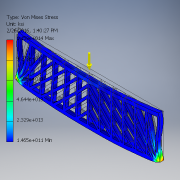
# Autodesk Inventor part: Haupt
Saved by Autodesk Inventor 2016 (Build 200138000, 138)
## iProperties
Created: 2016-02-25
Part Number: Haupt
Material: ABS Plastic
Document SubType Name: Modeling
Designer: 1750019
Density: 1.06 g/cm^3
Appearance: Smooth - White
Mass: 7.89342 g
Surface Area: 110.255 cm^2
Volume: 7.44663 cm^3
Author: 1750019
Autodesk Inventor part; units mm, degrees
ref_plane "YZ Plane" through (0, 0, 0) normal (1, 0, 0) x (0, 1, 0)
ref_plane "XZ Plane" through (0, 0, 0) normal (0, 1, 0) x (-1, 0, 0)
ref_plane "XY Plane" through (0, 0, 0) normal (0, 0, 1) x (1, 0, 0)
sketch "Sketch1" plane through (0, 0, 0) normal (0, 0, 1) x (1, 0, 0)
  line L0 (0, 0) -> (132.2917, 0) construction
  line L1 (132.2917, 0) -> (132.2917, -49.2125) construction
  line L2 (132.2917, -49.2125) -> (0, -49.2125) construction
  line L3 (0, -49.2125) -> (0, 0) construction
  line L4 (0, 0) -> (3.0776, 0) construction
  line L5 (3.0776, -2.3503) -> (3.0776, 0) construction
  line L6 (3.0776, -2.3503) -> (3.0776, -39.2903)
  line L7 (3.0776, -39.2903) -> (129.7257, -39.2903)
  line L8 (129.7257, -39.2903) -> (129.7257, -2.3503)
  line L9 (129.7257, -2.3503) -> (3.0776, -2.3503)
  line L10 (127.7764, -5.4053) -> (127.7764, -32.6911)
  line L11 (4.5608, -34.0848) -> (4.5608, -5.4053)
  line L12 (6.1422, -36.2512) -> (13.5226, -11.3064)
  line L13 (4.5608, -34.0848) -> (13.281, -5.4053)
  line L14 (57.0276, -34.9071) -> (65.3338, -26.3655)
  line L15 (58.4098, -36.2512) -> (65.3338, -29.1311)
  line L16 (127.7764, -32.6911) -> (119.3002, -5.4053)
  line L17 (119.3002, -12.0971) -> (126.3383, -36.2512)
  line L18 (74.4483, -36.2512) -> (67.1832, -28.7272)
  line L19 (75.8144, -34.9321) -> (67.1832, -25.9933)
  line L20 (4.5608, -5.4053) -> (13.281, -5.4053)
  line L21 (13.5226, -11.3064) -> (13.5226, -23.6805)
  line L22 (8.2509, -36.2512) -> (13.5226, -27.2721)
  line L23 (15.2246, -24.3731) -> (23.8802, -9.6304)
  line L24 (6.1422, -36.2512) -> (13.5226, -23.6805)
  line L25 (15.233, -20.7672) -> (23.8802, -6.0388)
  line L26 (8.2509, -36.2512) -> (13.5226, -29.8719)
  line L27 (10.6077, -36.2512) -> (13.5226, -32.7238)
  line L28 (13.5226, -36.2512) -> (10.6077, -36.2512)
  line L29 (17.7071, -36.2512) -> (23.8802, -29.7591)
  line L30 (23.8802, -36.2512) -> (23.8802, -29.7591)
  line L31 (25.4476, -28.1107) -> (25.4476, -36.2512)
  line L32 (15.1971, -36.2512) -> (23.8802, -27.1194)
  line L33 (23.8802, -36.2512) -> (17.7071, -36.2512)
  line L34 (25.569, -36.2512) -> (25.4476, -36.2512)
  line L35 (13.5226, -27.2721) -> (13.5226, -29.8719)
  line L36 (13.5226, -32.7238) -> (13.5226, -36.2512)
  line L37 (15.1971, -36.2512) -> (15.21, -30.6819)
  line L38 (15.2167, -27.8219) -> (15.2246, -24.3731)
  line L39 (15.233, -20.7672) -> (15.2686, -5.4053)
  line L40 (23.8802, -6.0388) -> (23.8802, -5.4053)
  line L41 (15.2686, -5.4053) -> (23.8802, -5.4053)
  line L42 (15.2167, -27.8219) -> (23.8802, -17.3381)
  line L43 (25.4476, -15.4414) -> (33.7411, -5.4053)
  line L44 (23.8802, -27.1194) -> (23.8802, -20.19)
  line L45 (23.8802, -17.3381) -> (23.8802, -9.6304)
  line L46 (25.4476, -5.4053) -> (25.4476, -15.4414)
  line L47 (25.4476, -18.2933) -> (25.4476, -25.471)
  line L48 (15.21, -30.6819) -> (23.8802, -20.19)
  line L49 (33.7411, -36.2512) -> (33.7411, -30.6389)
  line L50 (35.7136, -36.2512) -> (35.7136, -28.6156)
  line L51 (25.569, -36.2512) -> (33.7411, -27.8688)
  line L52 (28.2696, -36.2512) -> (33.7411, -30.6389)
  line L53 (33.7411, -36.2512) -> (28.2696, -36.2512)
  line L54 (33.7411, -27.8688) -> (33.7411, -19.3886)
  line L55 (33.7411, -16.7489) -> (33.7411, -8.2573)
  line L56 (25.4476, -25.471) -> (33.7411, -16.7489)
  line L57 (35.7136, -14.6745) -> (44.5272, -5.4053)
  line L58 (35.7136, -25.8455) -> (35.7136, -17.3142)
  line L59 (35.7136, -14.6745) -> (35.7136, -5.4053)
  line L60 (25.4476, -28.1107) -> (33.7411, -19.3886)
  line L61 (35.7136, -17.3142) -> (44.5272, -8.045)
  line L62 (25.4476, -18.2933) -> (33.7411, -8.2573)
  line L63 (25.4476, -5.4053) -> (33.7411, -5.4053)
  line L64 (35.7136, -5.4053) -> (44.5272, -5.4053)
  line L65 (35.7136, -25.8455) -> (44.5272, -16.805)
  line L66 (46.4045, -14.8793) -> (55.1798, -5.8781)
  line L67 (35.7136, -28.6156) -> (44.5272, -19.5751)
  line L68 (46.4045, -17.6495) -> (55.1798, -8.6483)
  line L69 (46.4045, -14.8793) -> (46.4045, -5.4053)
  line L70 (44.5272, -8.045) -> (44.5272, -16.805)
  line L71 (36.0978, -36.2512) -> (44.5272, -27.6711)
  line L72 (44.5272, -19.5751) -> (44.5272, -27.6711)
  line L73 (44.5272, -30.4311) -> (44.5272, -36.2512)
  line L74 (46.4045, -34.3207) -> (46.4045, -28.5054)
  line L75 (46.4045, -25.7602) -> (46.4045, -17.6495)
  line L76 (38.8531, -36.2512) -> (44.5272, -30.4311)
  line L77 (55.1798, -27.8779) -> (55.1798, -36.2512)
  line L78 (47.0372, -36.2512) -> (55.1798, -27.8779)
  line L79 (57.0276, -25.9778) -> (65.3338, -17.4362)
  line L80 (57.0276, -25.9778) -> (57.0276, -34.9071)
  line L81 (46.4045, -34.3207) -> (55.1798, -25.2968)
  line L82 (57.0276, -23.3967) -> (65.3338, -14.8551)
  line L83 (44.5272, -36.2512) -> (38.8531, -36.2512)
  line L84 (36.0978, -36.2512) -> (35.7136, -36.2512)
  line L85 (55.1798, -36.2512) -> (47.0372, -36.2512)
  line L86 (65.3338, -36.2512) -> (58.4098, -36.2512)
  line L87 (65.3338, -29.1311) -> (65.3338, -36.2512)
  line L88 (67.1832, -28.7272) -> (67.1832, -36.2512)
  line L89 (65.3338, -17.4362) -> (65.3338, -26.3655)
  line L90 (67.1832, -17.0999) -> (67.1832, -25.9933)
  line L91 (55.1798, -8.6483) -> (55.1798, -16.8279)
  line L92 (55.1798, -19.5042) -> (55.1798, -25.2968)
  line L93 (46.4045, -25.7602) -> (55.1798, -16.8279)
  line L94 (57.0276, -14.9471) -> (65.3338, -6.4923)
  line L95 (57.0276, -5.4053) -> (57.0276, -14.9471)
  line L96 (57.0276, -17.6089) -> (57.0276, -23.3967)
  line L97 (46.4045, -28.5054) -> (55.1798, -19.5042)
  line L98 (57.0276, -17.6089) -> (65.3338, -9.0889)
  line L99 (46.4045, -5.4053) -> (55.1798, -5.4053)
  line L100 (55.1798, -5.8781) -> (55.1798, -5.4053)
  line L101 (65.3338, -5.4053) -> (65.3338, -6.4923)
  line L102 (65.3338, -9.0889) -> (65.3338, -14.8551)
  line L103 (57.0276, -5.4053) -> (65.3338, -5.4053)
  line L104 (67.1832, -5.4053) -> (67.1832, -5.9402)
  line L105 (67.1832, -8.6483) -> (67.1832, -14.7032)
  line L106 (74.4483, -36.2512) -> (67.1832, -36.2512)
  line L107 (67.1832, -17.0999) -> (75.8144, -26.0387)
  line L108 (77.2599, -27.5358) -> (85.6755, -36.2512)
  line L109 (77.2599, -27.5358) -> (77.2599, -36.2512)
  line L110 (86.1387, -34.2095) -> (77.2599, -25.0728)
  line L111 (75.8144, -23.5852) -> (67.1832, -14.7032)
  line L112 (75.8144, -26.0387) -> (75.8144, -34.9321)
  line L113 (75.8144, -5.4053) -> (75.8144, -14.879)
  line L114 (75.8144, -17.5871) -> (75.8144, -23.5852)
  line L115 (67.1832, -8.6483) -> (75.8144, -17.5871)
  line L116 (75.8144, -14.879) -> (67.1832, -5.9402)
  line L117 (77.2599, -7.7529) -> (77.2599, -16.376)
  line L118 (77.2599, -19.0842) -> (77.2599, -25.0728)
  line L119 (67.1832, -5.4053) -> (75.8144, -5.4053)
  line L120 (87.9804, -5.4053) -> (87.9804, -5.8429)
  line L121 (86.1384, -5.4523) -> (86.1384, -14.5891)
  line L122 (77.2597, -5.4523) -> (86.1384, -14.5891)
  line L123 (77.2599, -7.7529) -> (86.1387, -16.8896)
  line L124 (87.9804, -8.3771) -> (87.9804, -16.5313)
  line L125 (96.4511, -36.2512) -> (87.9804, -27.4786)
  line L126 (86.1387, -25.5712) -> (77.2599, -16.376)
  line L127 (86.1387, -16.8896) -> (86.1387, -25.5712)
  line L128 (86.1387, -28.2794) -> (86.1387, -34.2095)
  line L129 (87.9804, -18.7849) -> (87.9804, -27.4786)
  line L130 (87.9804, -30.1867) -> (87.9804, -36.2512)
  line L131 (77.2599, -19.0842) -> (86.1387, -28.2794)
  line L132 (87.9804, -30.1867) -> (93.8362, -36.2512)
  line L133 (85.6755, -36.2512) -> (77.2599, -36.2512)
  line L134 (93.8362, -36.2512) -> (87.9804, -36.2512)
  line L135 (87.9804, -18.7849) -> (96.4511, -27.5018)
  line L136 (98.2148, -29.3167) -> (104.9535, -36.2512)
  line L137 (96.4511, -27.5018) -> (96.4511, -36.2512)
  line L138 (87.9804, -16.5313) -> (96.4511, -25.2482)
  line L139 (98.2148, -27.0631) -> (107.1434, -36.2512)
  line L140 (96.4511, -17.0941) -> (87.9804, -8.3771)
  line L141 (96.4511, -5.4053) -> (96.4511, -14.5598)
  line L142 (96.4511, -17.0941) -> (96.4511, -25.2482)
  line L143 (96.4511, -14.5598) -> (87.9804, -5.8429)
  line L144 (98.2148, -6.5789) -> (98.2148, -16.3747)
  line L145 (87.9804, -5.4053) -> (96.4511, -5.4053)
  line L146 (98.2148, -18.909) -> (98.2148, -27.0631)
  line L147 (98.2148, -29.3167) -> (98.2148, -36.2512)
  line L148 (104.9535, -36.2512) -> (98.2148, -36.2512)
  line L149 (107.1434, -28.0971) -> (107.1434, -36.2512)
  line L150 (117.53, -36.2512) -> (109.1269, -27.6039)
  line L151 (107.1434, -25.5628) -> (98.2148, -16.3747)
  line L152 (115.0673, -36.2512) -> (109.1269, -30.1382)
  line L153 (107.1434, -28.0971) -> (98.2148, -18.909)
  line L154 (109.1269, -30.1382) -> (109.1269, -36.2512)
  line L155 (107.1434, -17.7353) -> (98.2148, -6.5789)
  line L156 (107.1434, -15.2375) -> (99.2746, -5.4053)
  line L157 (109.1269, -9.6657) -> (109.1269, -17.7159)
  line L158 (109.1269, -20.2137) -> (109.1269, -27.6039)
  line L159 (107.1434, -5.4053) -> (107.1434, -15.2375)
  line L160 (107.1434, -17.7353) -> (107.1434, -25.5628)
  line L161 (99.2746, -5.4053) -> (107.1434, -5.4053)
  line L162 (109.1269, -5.4053) -> (117.53, -5.4053)
  line L163 (119.3002, -5.4053) -> (127.7764, -5.4053)
  line L164 (109.1269, -5.4053) -> (117.53, -20.4652)
  line L165 (119.3002, -23.6377) -> (126.3383, -36.2512)
  line L166 (117.53, -5.4053) -> (117.53, -20.4652)
  line L167 (119.3002, -12.0971) -> (119.3002, -23.6377)
  line L168 (119.3002, -27.8981) -> (119.3002, -36.2512)
  line L169 (109.1269, -9.6657) -> (117.53, -24.7256)
  line L170 (119.3002, -27.8981) -> (123.9611, -36.2512)
  line L171 (117.53, -24.7256) -> (117.53, -28.2156)
  line L172 (117.53, -30.7133) -> (117.53, -36.2512)
  line L173 (123.9611, -36.2512) -> (119.3002, -30.4274)
  line L174 (117.53, -28.2156) -> (109.1269, -17.7159)
  line L175 (121.9621, -36.2512) -> (119.3002, -32.9252)
  line L176 (117.53, -30.7133) -> (109.1269, -20.2137)
  line L177 (115.0673, -36.2512) -> (109.1269, -36.2512)
  line L178 (121.9621, -36.2512) -> (119.3002, -36.2512)
  line L179 (77.2597, -5.4523) -> (86.1384, -5.4523)
  dimension "d165" = 17.257
  dimension "d166" = 16.245
  dimension "d167" = 29.161
  dimension "d168" = 38.671
  dimension "d169" = 44.18
  dimension "d170" = 43.997
  dimension "d171" = 44.2
  dimension "d172" = 44.492
  dimension "d173" = 44.272
  dimension "d174" = 44.492
  dimension "d175" = 43.557
  dimension "d176" = 44.492
  dimension "d177" = 39.569
  dimension "d178" = 30.418
  dimension "d179" = 0.133
  dimension "d180" = 0.133
  dimension "d181" = 0.133
  dimension "d182" = 16.482
  dimension "d183" = 16.912
  dimension "d184" = 2.566
  dimension "d185" = 4.5152
  dimension "d186" = 12.9915
  dimension "d187" = 12.9915
  dimension "d188" = 14.7616
  dimension "d189" = 14.7616
  dimension "d190" = 14.7616
  dimension "d191" = 23.1647
  dimension "d192" = 23.1647
  dimension "d193" = 23.1647
  dimension "d194" = 25.1483
  dimension "d195" = 25.1483
  dimension "d196" = 25.1483
  dimension "d197" = 34.0769
  dimension "d198" = 34.0769
  dimension "d199" = 34.0769
  dimension "d200" = 35.8405
  dimension "d201" = 35.8405
  dimension "d202" = 35.8405
  dimension "d203" = 44.3113
  dimension "d204" = 44.3113
  dimension "d205" = 44.3113
  dimension "d206" = 44.3113
  dimension "d207" = 46.153
  dimension "d208" = 46.153
  dimension "d209" = 46.1532
  dimension "d210" = 55.0318
  dimension "d211" = 55.0318
  dimension "d212" = 55.0318
  dimension "d213" = 56.4773
  dimension "d214" = 56.4773
  dimension "d215" = 56.4773
  dimension "d216" = 65.1085
  dimension "d217" = 65.1085
  dimension "d218" = 65.1085
  dimension "d219" = 65.1085
  dimension "d220" = 66.9578
  dimension "d221" = 66.9578
  dimension "d222" = 66.9578
  dimension "d223" = 66.9578
  dimension "d224" = 75.2641
  dimension "d225" = 75.2641
  dimension "d226" = 75.2641
  dimension "d227" = 77.1118
  dimension "d228" = 77.1118
  constraints: 895 perpendicular, 352 end point, 114 parallel, 5 point on line, 1 horizontal, 2 other
  measures "d165" angle of L1 L16
  measures "d166" angle of L1 L17
  measures "d167" angle of L1 L165
  measures "d168" angle of L1 L173
  measures "d169" angle of L1 L150
  measures "d170" angle of L1 L125
  measures "d171" angle of L1 L15
  measures "d172" angle of L1 L94
  measures "d173" angle of L1 L98
  measures "d174" angle of L1 L93
  measures "d175" angle of L1 L61
  measures "d176" angle of L1 L71
  measures "d177" angle of L1 L43
  measures "d178" angle of L1 L23
  measures "d179" angle of L1 L39
  measures "d180" angle of L1 L38
  measures "d181" angle of L1 L37
  measures "d182" angle of L1 L12
  measures "d183" angle of L1 L13
  measures "d184" distance between parallel lines of L1 L8
  measures "d185" distance between parallel lines of L1 L10
  measures "d186" distance between parallel lines of L1 L167
  measures "d187" distance between parallel lines of L1 L168
  measures "d188" distance between parallel lines of L1 L166
  measures "d189" distance between parallel lines of L1 L171
  measures "d190" distance between parallel lines of L1 L172
  measures "d191" distance between parallel lines of L1 L157
  measures "d192" distance between parallel lines of L1 L158
  measures "d193" distance between parallel lines of L1 L154
  measures "d194" distance between parallel lines of L1 L159
  measures "d195" distance between parallel lines of L1 L160
  measures "d196" distance between parallel lines of L1 L149
  measures "d197" distance between parallel lines of L1 L144
  measures "d198" distance between parallel lines of L1 L146
  measures "d199" distance between parallel lines of L1 L147
  measures "d200" distance between parallel lines of L1 L141
  measures "d201" distance between parallel lines of L1 L142
  measures "d202" distance between parallel lines of L1 L137
  measures "d203" distance between parallel lines of L1 L120
  measures "d204" distance between parallel lines of L1 L124
  measures "d205" distance between parallel lines of L1 L129
  measures "d206" distance between parallel lines of L1 L130
  measures "d207" distance between parallel lines of L1 L127
  measures "d208" distance between parallel lines of L1 L128
  measures "d209" distance between parallel lines of L1 L121
  measures "d210" distance between parallel lines of L1 L117
  measures "d211" distance between parallel lines of L1 L118
  measures "d212" distance between parallel lines of L1 L109
  measures "d213" distance between parallel lines of L1 L113
  measures "d214" distance between parallel lines of L1 L114
  measures "d215" distance between parallel lines of L1 L112
  measures "d216" distance between parallel lines of L1 L104
  measures "d217" distance between parallel lines of L1 L105
  measures "d218" distance between parallel lines of L1 L90
  measures "d219" distance between parallel lines of L1 L88
  measures "d220" distance between parallel lines of L1 L101
  measures "d221" distance between parallel lines of L1 L102
  measures "d222" distance between parallel lines of L1 L89
  measures "d223" distance between parallel lines of L1 L87
  measures "d224" distance between parallel lines of L1 L95
  measures "d225" distance between parallel lines of L1 L96
  measures "d226" distance between parallel lines of L1 L80
  measures "d227" distance between parallel lines of L1 L100
  measures "d228" distance between parallel lines of L1 L91
extrude "Extrusion1" add sketch "Sketch1" along normal blind 3.175
body "Solid1"
